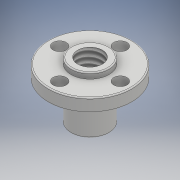
# Autodesk Inventor part: CastanhaTR8
Saved by Autodesk Inventor 2018 (Build 220112000, 112)
## iProperties
Created: 2018-09-20
Part Number: CastanhaTR8
Material: Genérico
Document SubType Name: Modeling
Designer: Georgines
Density: 1 g/cm^3
Appearance: Padrão
Author: Georgines
Autodesk Inventor part; units mm, degrees
ref_plane "YZ Plane" through (0, 0, 0) normal (1, 0, 0) x (0, 1, 0)
ref_plane "XZ Plane" through (0, 0, 0) normal (0, 1, 0) x (-1, 0, 0)
ref_plane "XY Plane" through (0, 0, 0) normal (0, 0, 1) x (1, 0, 0)
sketch "Esboço1" plane through (0, 0, 0) normal (0, 0, 1) x (1, 0, 0)
  circle A0 centre (0, 0) radius 11
  dimension "d0" = 22
  constraints: 1 centre point, 1 coincident
  measures "d0" diameter of A0
extrude "Extrusão1" add sketch "Esboço1" along normal blind 3.5
sketch "Esboço2" plane through (0, 0, 3.5) normal (0, 0, 1) x (1, 0, 0)
  circle A0 centre (0, 0) radius 5
  dimension "d3" = 10
  constraints: 1 centre point, 1 coincident
  measures "d3" diameter of A0
extrude "Extrusão2" add sketch "Esboço2" along normal blind 1.5
sketch "Esboço3" plane through (0, 0, 0) normal (0, 0, -1) x (-1, 0, 0)
  circle A0 centre (0, 0) radius 5
  dimension "d6" = 10
  constraints: 1 centre point, 1 coincident
  measures "d6" diameter of A0
extrude "Extrusão3" add sketch "Esboço3" along normal blind 10
sketch "Esboço4" plane through (0, 0, 3.5) normal (0, 0, 1) x (1, 0, 0)
  circle A0 centre (0, 0) radius 8 construction
  circle A1 centre (-8, 0) radius 1 construction
  circle A2 centre (0, -8) radius 1 construction
  circle A3 centre (0, 0) radius 8 construction
  circle A4 centre (8, 0) radius 1 construction
  circle A5 centre (0, 0) radius 8 construction
  circle A6 centre (0, 8) radius 1 construction
  circle A7 centre (0, 0) radius 8 construction
  dimension "d9" = 16
  dimension "d10" = 2
  dimension "d13" = 360
  constraints: 4 centre point, 3 coincident, 2 horizontal alignment, 2 vertical alignment, 23 other
  measures "d10" diameter of A1
hole "Furo1" at (-8, 0, 3.5) at (0, -8, 3.5) at (8, 0, 3.5) at (0, 8, 3.5) direction (0, 0, -1) diameter 3.5 end through all
fillet "Arredondamento1" radius 0.3 4 edges at (-11, 0, 3.5) (-11, 0, 0) (5, 0, -10) (-5, 0, 5)
sketch "Esboço5" plane through (0, 0, 5) normal (0, 0, 1) x (1, 0, 0)
  circle A0 centre (0, 0) radius 1.5 construction
  dimension "d23" = 3
  constraints: 1 centre point, 1 coincident
  measures "d23" diameter of A0
hole "Furo2" at (0, 0, 5) direction (0, 0, -1) diameter 6.5 end through all thread size "TR8x1.5" class "7H" standard "ISO Metric Trapezoidal Threads"
